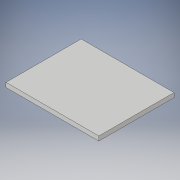
# Autodesk Inventor part: ita
Saved by Autodesk Inventor 2019.3 (Build 233278000, 278)
## iProperties
Created: 2018-12-23
Part Number: ita
Material: 一般
Document SubType Name: Modeling
Designer: masaya
Density: 1 g/cm^3
Appearance: 既定
Author: masaya
Autodesk Inventor part; units mm, degrees
ref_plane "YZ Plane" through (0, 0, 0) normal (1, 0, 0) x (0, 1, 0)
ref_plane "XZ Plane" through (0, 0, 0) normal (0, 1, 0) x (-1, 0, 0)
ref_plane "XY Plane" through (0, 0, 0) normal (0, 0, 1) x (1, 0, 0)
sketch "スケッチ1" plane through (0, 0, 0) normal (0, 1, 0) x (-1, 0, 0)
  line L0 (0, 0) -> (2100, 0)
  line L1 (2100, 0) -> (2100, 1700)
  line L2 (2100, 1700) -> (0, 1700)
  line L3 (0, 1700) -> (0, 0)
  dimension "d0" = 2100
  dimension "d2" = 1700
  constraints: 8 end point, 2 parallel, 1 horizontal, 1 perpendicular
  measures "d0" distance of L2.end L1.end
  measures "d2" distance of L2.end L0.start
extrude "押し出し1" add sketch "スケッチ1" along normal blind 100
